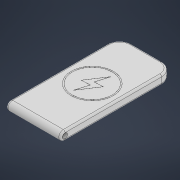
# Autodesk Inventor part: WirelessChargerBase
Saved by Autodesk Inventor 2021 (Build 250183000, 183)
## iProperties
Created: 2021-01-30
Part Number: WirelessChargerBase
Material: Generic
Document SubType Name: Modeling
Designer: argon
Density: 1 g/cm^3
Appearance: Default
Author: argon
Autodesk Inventor part; units mm, degrees
ref_plane "YZ Plane" through (0, 0, 0) normal (1, 0, 0) x (0, 1, 0)
ref_plane "XZ Plane" through (0, 0, 0) normal (0, 1, 0) x (-1, 0, 0)
ref_plane "XY Plane" through (0, 0, 0) normal (0, 0, 1) x (1, 0, 0)
sketch "Sketch1" plane through (0, 0, 0) normal (1, 0, 0) x (0, 1, 0)
  circle A0 centre (0, 0) radius 7.5
  line L0 (7.5, 0) -> (7.5, -180)
  line L1 (-7.5, 0) -> (-7.5, -180)
  line L2 (-7.5, -180) -> (7.5, -180)
  circle A1 centre (0, 0) radius 4
  dimension "d0" = 15
  dimension "d1" = 180
  dimension "d2" = 8
  constraints: 6 end point, 2 centre point, 2 coincident, 2 point on circle, 2 point on line, 2 tangent, 2 vertical, 1 horizontal
  measures "d0" diameter of A0
  measures "d1" distance of L0.start L0.end
  measures "d2" diameter of A1
extrude "Extrusion1" add sketch "Sketch1" along normal blind 90
fillet "Fillet1" radius 3 8 edges at (90, 0, 7.5) (90, 7.5, -90) (90, -7.5, -90) (0, 0, 7.5) (0, -7.5, -90) (0, 7.5, -90) (45, 7.5, -180) (45, -7.5, -180)
fillet "Fillet1" radius 20 2 edges at (90, 0, -180) (0, 0, -180)
sketch "Sketch2" plane through (3, 7.5, 0) normal (0, 1, 0) x (1, 0, 0)
  circle A0 centre (42, 90) radius 35
  line L0 (0, 0) -> (84, 0) projected
  line L1 (84, 160) -> (84, 0) projected
  circle A1 centre (42, 90) radius 33
  circle A2 centre (42, 90) radius 26 construction
  line L2 (47.8487, 115.3336) -> (28.2097, 85.5193)
  line L3 (48.5399, 83.4738) -> (36.1513, 64.6664)
  line L4 (36.1513, 64.6664) -> (55.7903, 94.4807)
  line L5 (55.7903, 94.4807) -> (41.4332, 93.7457)
  line L6 (41.4332, 93.7457) -> (47.8487, 115.3336)
  line L7 (47.8487, 115.3336) -> (36.1513, 64.6664) construction
  line L8 (-3, 160) -> (-3, 0) projected
  line L9 (28.2097, 85.5193) -> (55.7903, 94.4807) construction
  line L10 (28.2097, 85.5193) -> (42.5668, 86.2543)
  line L11 (42.5668, 86.2543) -> (36.1513, 64.6664)
  line L12 (41.4332, 93.7457) -> (42.5668, 86.2543) construction
  point P0 (42, 0)
  point P1 (84, 80)
  dimension "d7" = 10
  dimension "d8" = 70
  dimension "d9" = 2
  dimension "d10" = 7
  dimension "d27" = 13
  dimension "d35" = 72
  dimension "d42" = 29
  constraints: 20 end point, 5 midpoint, 3 centre point, 2 coincident, 2 equal length, 2 parallel, 2 point on circle, 1 vertical alignment
  measures "d7" vertical distance of point (84, 80) A0.centre
  measures "d8" diameter of A0
  measures "d9" radial gap between concentric circles of A0 A1
  measures "d10" radial gap between concentric circles of A1 A2
  measures "d27" angle of L8 L7
  measures "d35" angle of L8 L9
  measures "d42" distance of L2.end L4.end
extrude "Extrusion2" add sketch "Sketch2" along normal blind 0.1
sketch "Sketch3" plane through (70, 4.5, -180) normal (0, 0, -1) x (-1, 0, 0)
  line L0 (37, -7) -> (13, -7)
  line L1 (13, -7) -> (13, -2)
  line L2 (13, -2) -> (37, -2)
  line L3 (37, -2) -> (37, -7)
  line L4 (37, -7) -> (13, -2) construction
  line L5 (13, -7) -> (37, -2) construction
  line L6 (50, -9) -> (0, -9) projected
  line L7 (-20, -8.5) -> (-20, -0.5) projected
  point P0 (70, -4.5)
  point P1 (25, -4.5)
  point P2 (25, -9)
  point P3 (-20, -4.5)
  dimension "d52" = 5
  dimension "d53" = 24
  constraints: 12 end point, 4 midpoint, 2 parallel, 1 horizontal, 1 horizontal alignment, 1 perpendicular, 1 vertical alignment
  measures "d52" distance of L2.end L0.start
  measures "d53" distance of L0.start L0.end
extrude "Extrusion3" cut sketch "Sketch3" against normal blind 20
fillet "Fillet2" radius 1 4 edges at (45, -2.5, -180) (33, 0, -180) (57, 0, -180) (45, 2.5, -180)
fillet "Fillet3" radius 1 4 edges at (45, -2.5, -160) (33, 0, -160) (45, 2.5, -160) (57, 0, -160)
body "Solid1"
